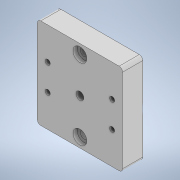
# Autodesk Inventor part: ADAPTER_EOM14.7GHz_new
Saved by Autodesk Inventor 2020 (Build 240168000, 168)
## iProperties
Created: 2021-07-16
Part Number: ADAPTER_EOM14.7GHz_new
Material: Generic
Document SubType Name: Modeling
Designer: paige
Density: 1 g/cm^3
Appearance: Default
Author: paige
Autodesk Inventor part; units mm, degrees
ref_plane "YZ Plane" through (0, 0, 0) normal (1, 0, 0) x (0, 1, 0)
ref_plane "XZ Plane" through (0, 0, 0) normal (0, 1, 0) x (-1, 0, 0)
ref_plane "XY Plane" through (0, 0, 0) normal (0, 0, 1) x (1, 0, 0)
sketch "Sketch1" plane through (0, 0, 0) normal (0, 0, 1) x (1, 0, 0)
  line L0 (-24.5, 26) -> (24.5, 26)
  line L1 (24.5, 26) -> (24.5, -26)
  line L2 (24.5, -26) -> (-24.5, -26)
  line L3 (-24.5, -26) -> (-24.5, 26)
  point P0 (0, 0)
  dimension "d0" = 52
  dimension "d1" = 26
  dimension "d2" = 49
  dimension "d3" = 24.5
  constraints: 8 end point, 2 parallel, 1 horizontal, 1 perpendicular
  measures "d0" distance of L2.end L0.start
  measures "d1" distance from line of L0 point (0, 0)
  measures "d2" distance of L1.end L2.end
  measures "d3" distance from line of L1 point (0, 0)
extrude "Extrusion1" add sketch "Sketch1" along normal blind 11.55
sketch "Sketch3" plane through (0, 0, 11.55) normal (0, 0, 1) x (1, 0, 0)
  line L0 (-24.5, -26) -> (24.5, -26) projected
  line L1 (0, -26) -> (0, -20.5)
  line L2 (24.5, 26) -> (-24.5, 26) projected
  line L3 (0, 26) -> (0, 20.5)
  point P0 (0, 0)
  point P1 (0, 0)
  dimension "d13" = 5.5
  dimension "d14" = 20.5
  dimension "d15" = 5.5
  dimension "d16" = 20.5
  constraints: 4 end point, 3 coincident, 2 midpoint, 2 vertical, 1 other
  measures "d13" distance of L1.start L1.end
  measures "d14" distance of point (0, 0) L1.end
  measures "d15" distance of L3.start L3.end
  measures "d16" distance of L3.end point (0, 0)
hole "Hole1" at (0, 20.5, 11.55) at (0, -20.5, 11.55) direction (0, 0, -1) diameter 4.305 depth 12.3 counterbore diameter 7.938 counterbore depth 2.4 clearance for "Socket Head Cap Screw" size "#8" standard "Ansi Unified Screw Threads"
sketch "Sketch5" plane through (0, 0, 0) normal (0, 0, -1) x (-1, 0, 0)
  line L0 (-24.5, 26) -> (24.5, 26) projected
  line L1 (24.5, 26) -> (24.5, -26) projected
  point P0 (0, 0)
  point P1 (0, 0)
  dimension "d31" = 26
  dimension "d32" = 24.5
  constraints: 1 coincident
  measures "d31" distance from line of L0 point (0, 0)
  measures "d32" distance from line of L1 point (0, 0)
hole "Hole3" at (0, 0, 0) direction (0, 0, 1) diameter 4.5 depth 11.8 counterbore diameter 8 counterbore depth 4 clearance for "Socket Head Cap Screw" size "M4" standard "Ansi Metric M Profile"
fillet "Fillet1" radius 2 4 edges at (-24.5, -26, 5.775) (-24.5, 26, 5.775) (24.5, -26, 5.775) (24.5, 26, 5.775)
sketch "Sketch7" plane through (-24.5, -24, 0) normal (-1, 0, 0) x (0, 0, 1)
  circle A0 centre (-12.35, 24) radius 12.7
  point P0 (0, 24)
  dimension "d57" = 25.4
  dimension "d58" = 12.35
  constraints: 1 centre point
  measures "d57" diameter of A0
  measures "d58" distance of point (0, 24) A0.centre
extrude "Extrusion3" cut sketch "Sketch7" against normal blind 50
sketch "Sketch10" plane through (0, 0, 0) normal (0, 0, -1) x (-1, 0, 0)
  circle A0 centre (0, 0) radius 1.621
  line L0 (0, 0) -> (-18.5, 0)
  line L1 (-18.5, 0) -> (-18.5, -7.5)
  line L2 (-18.5, -7.5) -> (0, -7.5)
  line L3 (0, -7.5) -> (0, 0)
  point P0 (-18.5, 7.5)
  point P1 (18.5, 7.5)
  point P2 (18.5, -7.5)
  dimension "d77" = 18.5
  dimension "d78" = 7.5
  dimension "d79" = 18.5
  dimension "d80" = 37
  dimension "d81" = 18.5
  dimension "d82" = 7.5
  dimension "d83" = 7.5
  dimension "d84" = 7.5
  constraints: 8 end point, 2 parallel, 1 centre point, 1 coincident, 1 horizontal, 1 perpendicular
  measures "d77" distance of L1.end L2.end
  measures "d78" distance of L0.end L1.end
  measures "d79" distance of L2.end point (18.5, -7.5)
  measures "d80" distance of point (-18.5, 7.5) point (18.5, 7.5)
  measures "d81" horizontal distance of point (0, 0) point (18.5, 7.5)
  measures "d82" distance of L0.end point (-18.5, 7.5)
  measures "d83" vertical distance of point (0, 0) point (18.5, 7.5)
  measures "d84" vertical distance of point (0, 0) point (18.5, -7.5)
hole "Hole5" at (18.5, -7.5, 0) at (18.5, 7.5, 0) at (-18.5, 7.5, 0) at (-18.5, -7.5, 0) direction (0, 0, 1) diameter 2.9 end through all counterbore diameter 5.5 counterbore depth 7.5 clearance for "Socket Head Cap Screw" size "M2.5" standard "Ansi Metric M Profile"
equation "\"d1\" = 0.5 * d0"
equation "\"d3\" = 0.5 * d2"
equation "\"d15\" = d13"
equation "\"d79\" = d77"
equation "\"d80\" = 2 * d77"
equation "\"d81\" = d77"
equation "\"d82\" = d78"
equation "\"d83\" = d78"
equation "\"d84\" = d78"
body "Solid1"
